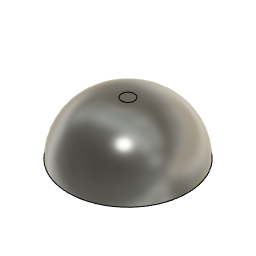
Topper - small dome v8 (Autodesk Fusion 360 design; units mm, degrees)
Autodesk Fusion 360 part; units mm, degrees
note: some values were not read from the file. Set by a fixed rule: which sketch regions a step uses.
sketch "Sketch1" plane through (0, 0, 0) normal (0, 1, 0) x (1, 0, 0)
  line L0 (0, 0) -> (7, 0)
  line L1 (0, 0) -> (0, -6.25)
  line L2 (0, -6.25) -> (0.75, -6.25)
  arc A0 (0.75, -6.25) -> (7, 0) centre (0.75, 0) ccw
  line L3 (7, 0) -> (7, -3.5) construction
  dimension "d1" = 7
  dimension "d7" = 0.75
  constraint coincident L0.start L1.start
  constraint horizontal L0
  constraint perpendicular L0 L1
  constraint perpendicular L1 L2
  constraint tangent L2 A0
  constraint perpendicular L0 L3
  constraint tangent A0 L3
  measures "d1" distance of L0.start L0.end
  measures "d7" distance of L1.end L2.end
revolve "Revolve1" add sketch "Sketch1" angle 360 about axis through (0, 0, 0) along (0, 0, 1)
sketch "Sketch2" plane through (0, 0, 0) normal (0, 0, -1) x (1, 0, 0)
  line L0 (-1.55, 1.05) -> (-1.55, -1.05)
  line L1 (1.55, 1.05) -> (1.55, -1.05)
  circle A0 centre (0, 0) radius 7
  line L2 (-0.55, 2.05) -> (0.55, 2.05)
  line L3 (-0.55, -2.05) -> (0.55, -2.05)
  arc A1 (-0.55, 2.05) -> (-1.55, 1.05) centre (-0.55, 1.05) ccw
  arc A2 (-1.55, -1.05) -> (-0.55, -2.05) centre (-0.55, -1.05) ccw
  arc A3 (0.55, -2.05) -> (1.55, -1.05) centre (0.55, -1.05) ccw
  arc A4 (1.55, 1.05) -> (0.55, 2.05) centre (0.55, 1.05) ccw
  point P0 (-1.55, 2.05)
  point P1 (1.55, 2.05)
  point P2 (1.55, -2.05)
  point P3 (0, 2.05)
  point P4 (1.55, 0)
  dimension "d8" = 3.1
  dimension "d9" = 4.1
  dimension "d10" = 1
  constraint vertical L0
  constraint vertical L1
  constraint perpendicular L1 L2
  constraint perpendicular L1 L3
  constraint vertical A0.centre P3
  constraint coincident L2 P3
  constraint coincident P0 L2
  constraint coincident P0 L0
  constraint tangent L2 A1
  constraint tangent L0 A1
  constraint tangent L0 A2
  constraint tangent L3 A2
  constraint equal A1 A2
  constraint coincident P2 L1
  constraint coincident P2 L3
  constraint tangent L1 A3
  constraint tangent L3 A3
  constraint equal A1 A3
  constraint coincident P1 L2
  constraint coincident P1 L1
  constraint tangent L2 A4
  constraint tangent L1 A4
  constraint equal A1 A4
  constraint midpoint L2 P3
  constraint midpoint L1 P4
  constraint horizontal A0.centre P4
  measures "d8" distance of P0 P1
  measures "d9" distance of P1 P2
  measures "d10" radius of A1
extrude "Extrude1" cut sketch "Sketch2" against normal blind 2.5 contours L0 L1 L2 L3 A1 A2 A3 A4
